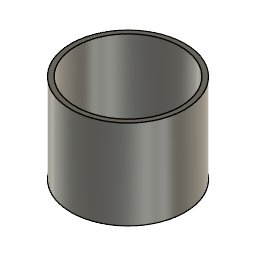
Final_flashpaper_chamber_outer (Autodesk Fusion 360 design; units mm, degrees)
part number: 2026-05-27-16-17-13-160
Autodesk Fusion 360 part; units mm, degrees
sketch "Sketch1" plane through (0, 0, 0) normal (0, 0, 1) x (1, 0, 0)
  circle A0 centre (0, 0) radius 18.2
  dimension "d5" = 36.4
  constraint coincident A0.centre origin
  measures "d5" diameter of A0
extrude "Extrude2" add sketch "Sketch1" along normal blind 28.5
shell "Shell2" thickness 1.5 removed faces 1 at (5.3342, 0.2875, 28.5)
